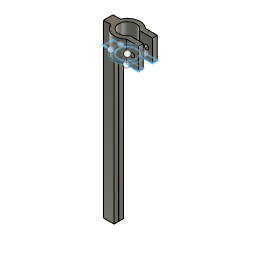
Frame v3 (Autodesk Fusion 360 archive; units mm, degrees)
design "Main Hold"
Autodesk Fusion 360 part; units mm, degrees
note: some values were not read from the file. Chosen so that the rebuilt part matches the saved one: which face or edge a step refers to. Set by a fixed rule: which sketch regions a step uses.
sketch "Sketch1" plane through (0, 0, 0) normal (0, 0, 1) x (1, 0, 0)
  line L0 (-6.8161, 4.6338) -> (-18.242, 4.6338)
  line L1 (8.001, -8.943) -> (19.5137, -8.943)
  line L2 (19.5137, -8.943) -> (19.5137, -4.443)
  line L3 (-18.242, -4.3662) -> (-6.9956, -4.3662)
  circle A0 centre (0.0069, -0.0041) radius 8.25
  arc A1 (-6.9956, -4.3662) -> (6.9609, -4.443) centre (0.0069, -0.0041) ccw
  line L4 (8.1435, 8.8053) -> (19.5137, 8.8053)
  line L5 (-11.0521, 4.6338) -> (-6.8161, 4.6338)
  line L6 (19.5137, 8.8053) -> (8.1435, 8.8053)
  line L7 (19.5137, -8.943) -> (19.5137, -4.443)
  arc A2 (-6.8161, 4.6338) -> (-6.9956, -4.3662) centre (0.0069, -0.0041) ccw
  line L8 (19.5137, 4.3053) -> (19.5137, 8.8053)
  line L9 (19.5137, 4.3053) -> (7.0419, 4.3053)
  circle A3 centre (0.0069, -0.0041) radius 12.0488
  line L10 (-18.242, 4.6338) -> (-18.242, -4.3662)
  line L11 (8.001, -8.943) -> (19.5137, -8.943)
  line L12 (19.5137, 4.3053) -> (19.5137, 8.8053)
  arc A4 (7.0419, 4.3053) -> (-6.8161, 4.6338) centre (0.0069, -0.0041) ccw
  line L13 (7.0419, 4.3053) -> (19.5137, 4.3053)
  line L14 (19.5137, -4.443) -> (6.9609, -4.443)
  line L15 (-11.0521, 4.6338) -> (-18.242, 4.6338)
  line L16 (-6.9956, -4.3662) -> (-11.1637, -4.3662)
  line L17 (-18.242, -4.3662) -> (-11.1637, -4.3662)
  line L18 (-18.242, 4.6338) -> (-18.242, -4.3662)
  line L19 (0.0069, -0.0041) -> (-18.242, -0.0041) construction
  line L20 (-8.2415, 0.1604) -> (-8.2415, -4.3662)
  line L21 (-8.2415, 0.1604) -> (-8.2415, 4.6355)
  line L22 (-8.2415, -4.3662) -> (-8.2415, 4.6355)
  dimension "d6" = 90
  constraint concentric A0 A2
  constraint concentric A0 A3
  constraint coincident L1.start L11.start
  constraint coincident L1.end L2.start
  constraint coincident L2.end L7.end
  constraint coincident L8.start L9.start
  constraint coincident L4.end L6.start
  constraint coincident L4.start L6.end
  constraint coincident L9.end A4.start
  constraint coincident L5.start L15.start
  constraint coincident L0.end L10.start
  constraint coincident L3.start L10.end
  constraint coincident L16.end L17.end
  constraint coincident A0.centre A1.centre
  constraint coincident L18 L19.end
  constraint perpendicular L18 L19
  constraint midpoint A2 L20.start
  constraint coincident L16 L20.end
  constraint coincident L3 L20.end
  constraint perpendicular L5 L21
  constraint perpendicular L0 L22
  measures "d6" angle of L19 L20
extrude "Extrude1" add sketch "Sketch1" along normal blind 20.5 contours L0 A0 L5 A2 L21 L22 | L0 A0 L5 L9 A3 A4 L13 L15 | L3 A0 A2 L16 L20 L22 | L0 L3 L5 A3 L15 L16 L17 L20 L21 L22 | L4 L6 L8 L9 A3 L12 L13 | L3 A0 A1 A3 L14 L16 L17 | L0 L3 A3 L10 L15 L17 L18 | L1 L2 L7 A3 L11 L14
sketch "Sketch2" plane through (0, 8.8053, 0) normal (0, 1, 0) x (-1, 0, 0)
  line L0 (-19.5137, 0) -> (-8.2268, 0)
  line L1 (-8.2268, 20.5) -> (-19.5137, 20.5)
  line L2 (-19.5137, 20.5) -> (-19.5137, 0)
  line L3 (-8.2268, 0) -> (-19.5137, 20.5) construction
  line L4 (-8.2268, 20.5) -> (-19.5137, 0) construction
  circle A0 centre (-13.8702, 10.25) radius 2
  line L5 (-8.2268, 0) -> (-8.2268, 20.5)
  dimension "d3" = 4
  constraint coincident L0.end L3.start
  constraint coincident L1.end L2.start
  constraint coincident L1.start L4.start
  constraint coincident L0.start L2.end
  constraint midpoint L4 A0.centre
  measures "d3" diameter of A0
extrude "Extrude2" cut sketch "Sketch2" against normal blind 39 contours A0
extrude "Extrude3" add sketch "Sketch1" against normal blind 141.5 contours L0 A0 L5 A2 L21 L22 | L3 A0 A2 L16 L20 L22 | L0 L3 L5 A3 L15 L16 L17 L20 L21 L22 | L0 L3 A3 L10 L15 L17 L18
extrude "Extrude4" cut sketch "Sketch1" against normal blind 144 contours L0 A0 L5 A2 L21 L22 | L3 A0 A2 L16 L20 L22
extrude "Extrude5" cut 2 faces at (-9.3904, -2.3691, -141.5) (-16.175, 0.1374, -141.5) along direction (0, 0, 1) blind 141
extrude "Extrude6" add 2 faces at (-9.3904, -2.3691, -0.5) (-16.175, 0.1374, -0.5) along direction (0, 0, -1) blind 141

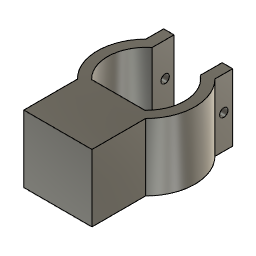
design "Motor Mount"
Autodesk Fusion 360 part; units mm, degrees
sketch "Sketch1" plane through (0, 0, 0) normal (0, 0, 1) x (1, 0, 0)
  arc A0 (7.9217, -8.3364) -> (7.9217, 8.3364) centre (0, 0) ccw
  line L0 (-7.1925, 15.5) -> (-10.2923, 15.5)
  line L1 (7.9217, -8.3364) -> (-7.9217, -8.3364)
  line L2 (7.1667, 15.5) -> (7.1667, 8.9938)
  line L3 (-10.2923, 15.5) -> (-10.2923, 10.2136)
  line L4 (10.2923, 15.5) -> (7.1667, 15.5)
  line L5 (7.9217, -8.3364) -> (-7.9217, -8.3364)
  line L6 (-10.2923, 15.5) -> (-10.2923, 10.2136)
  arc A1 (-10.2923, 10.2136) -> (-10.169, -10.3364) centre (0, 0) ccw
  line L7 (-7.1925, 15.5) -> (-7.1925, 8.9732)
  line L8 (10.2923, 10.2136) -> (10.2923, 15.5)
  arc A2 (-7.9217, 8.3364) -> (-7.9217, -8.3364) centre (0, 0) ccw
  circle A3 centre (0, 0) radius 11.5
  line L9 (-7.1925, 15.5) -> (-10.2923, 15.5)
  line L10 (10.2923, 10.2136) -> (10.2923, 15.5)
  line L11 (10.2923, 15.5) -> (7.1667, 15.5)
  arc A4 (10.169, -10.3364) -> (10.2923, 10.2136) centre (0, 0) ccw
  line L12 (10.169, -10.3364) -> (10.169, -26.3364)
  line L13 (-10.169, -10.3364) -> (-10.169, -26.3364)
  line L14 (-10.169, -26.3364) -> (10.169, -26.3364)
  dimension "d1" = 16
  dimension "d2" = 16
  constraint coincident L8.start L10.start
  constraint coincident L4.start L8.end
  constraint coincident L2.start L4.end
  constraint perpendicular L2 L4
  constraint coincident L0.start L7.start
  constraint coincident L0.end L3.start
  constraint coincident L3.end L6.end
  constraint perpendicular L0 L7
  constraint coincident A0.start L1.start
  constraint coincident L1.end L5.end
  constraint concentric A2 A3
  constraint coincident L2.end A3
  constraint vertical L2
  constraint coincident L7.end A3
  constraint vertical L7
  constraint vertical L12
  constraint vertical L13
  constraint perpendicular L12 L14
  measures "d1" distance of A4.start L12.end
  measures "d2" distance of A1.end L13.end
extrude "Extrude1" add sketch "Sketch1" along normal blind 20 contours L1 L5 A3 | A0 L0 L2 L3 L4 L6 A1 L7 L8 A2 A3 L9 L10 L11 A4 L12 L13 L14
sketch "Sketch2" plane through (10.2923, 0, 0) normal (1, 0, 0) x (0, 1, 0)
  line L0 (10.2136, 0) -> (15.5, 0)
  line L1 (15.5, 0) -> (15.5, 20)
  line L2 (15.5, 20) -> (10.2136, 20)
  line L3 (10.2136, 20) -> (10.2136, 0)
  line L4 (10.2136, 20) -> (15.5, 0) construction
  line L5 (10.2136, 0) -> (15.5, 20) construction
  circle A0 centre (12.8568, 10) radius 1.25
  dimension "d5" = 2.5
  constraint coincident L2.end L3.start
  constraint coincident L0.end L1.start
  constraint coincident L0.start L3.end
  constraint coincident L1.end L2.start
  constraint midpoint L5 A0.centre
  measures "d5" diameter of A0
extrude "Extrude2" cut sketch "Sketch2" against normal blind 21 contours A0

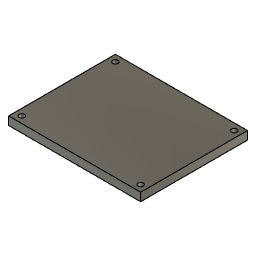
design "PCB Mount"
Autodesk Fusion 360 part; units mm, degrees
sketch "Sketch1" plane through (0, 0, 0) normal (0, 0, 1) x (1, 0, 0)
  circle A0 centre (36.1, -17.1) radius 1.65
  line L0 (-40.064, 43.7) -> (-40.064, -21.1)
  circle A1 centre (36.1, -17.1) radius 1.65
  circle A2 centre (-36.064, 39.7) radius 1.65
  line L1 (-40.064, -21.1) -> (40.1, -21.1)
  circle A3 centre (36.1, 39.7) radius 1.65
  circle A4 centre (-36.064, -17.1) radius 1.65
  line L2 (40.1, -21.1) -> (40.1, 43.7)
  circle A5 centre (-36.064, 39.7) radius 1.65
  line L3 (-40.064, -21.1) -> (-40.064, 43.7)
  circle A6 centre (36.1, 39.7) radius 1.65
  circle A7 centre (-36.064, -17.1) radius 1.65
  line L4 (40.1, 43.7) -> (40.1, -21.1)
  line L5 (40.1, 43.7) -> (-40.064, 43.7)
  constraint coincident L0.end L1.start
  constraint coincident L0.start L3.end
  constraint coincident L2.end L4.start
  constraint coincident L1.end L2.start
  constraint concentric A0 A1
  constraint concentric A4 A7
  constraint concentric A2 A5
  constraint concentric A3 A6
extrude "Extrude1" add sketch "Sketch1" along normal blind 5
